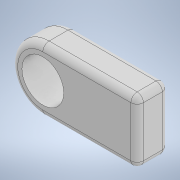
# Autodesk Inventor part: Part1
Saved by Autodesk Inventor 2021.1 (Build 251245010, 245A)
## iProperties
Created: 2024-03-27
Part Number: Part1
Material: Generic
Document SubType Name: Modeling
Designer: peter
Density: 1 g/cm^3
Appearance: Default
Author: peter
Autodesk Inventor part; units mm, degrees
ref_plane "YZ Plane" through (0, 0, 0) normal (1, 0, 0) x (0, 1, 0)
ref_plane "XZ Plane" through (0, 0, 0) normal (0, 1, 0) x (-1, 0, 0)
ref_plane "XY Plane" through (0, 0, 0) normal (0, 0, 1) x (1, 0, 0)
sketch "Sketch1" plane through (0, 0, 0) normal (0, 0, 1) x (1, 0, 0)
  circle A0 centre (0, 0) radius 6.65
  arc A1 (0, 10) -> (0, -10) centre (0, 0) ccw
  line L0 (0, 10) -> (30, 10)
  line L1 (30, 10) -> (30, -10)
  line L2 (30, -10) -> (0, -10)
  dimension "d0" = 13.3
  dimension "d2" = 20
  dimension "d3" = 30
  dimension "d4" = 20
  constraints: 6 end point, 2 centre point, 2 coincident, 2 point on circle, 2 tangent, 1 horizontal, 1 perpendicular
  measures "d0" diameter of A0
  measures "d2" diameter of A1
  measures "d3" distance of L0.start L0.end
  measures "d4" distance of L0.end L1.end
extrude "Extrusion1" add sketch "Sketch1" along normal blind 10
fillet "Fillet1" radius 2 10 edges at (30, 10, 5) (30, 0, 10) (-10, 0, 10) (15, -10, 10) (15, 10, 10) (-10, 0, 0) (15, -10, 0) (15, 10, 0) (30, 0, 0) (30, -10, 5)
body "Solid1"
